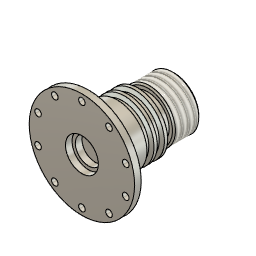
peer challenge (Autodesk Fusion 360 design; units mm, degrees)
Autodesk Fusion 360 part; units mm, degrees
sketch "Sketch1" plane through (0, 0, 0) normal (1, 0, 0) x (0, 0, -1)
  line L0 (0, 0) -> (0, 50.8)
  line L1 (0, 50.8) -> (6.35, 50.8)
  line L2 (6.35, 50.8) -> (6.35, 31.75)
  line L3 (6.35, 31.75) -> (9.525, 28.575)
  line L4 (9.525, 28.575) -> (34.1224, 28.575)
  line L5 (34.1224, 28.575) -> (35.9555, 25.4)
  line L6 (35.9555, 25.4) -> (39.1305, 25.4)
  line L7 (39.1305, 25.4) -> (40.9636, 28.575)
  line L8 (40.9636, 28.575) -> (44.1386, 28.575)
  line L9 (44.1386, 28.575) -> (45.9717, 25.4)
  line L10 (45.9717, 25.4) -> (49.1467, 25.4)
  line L11 (49.1467, 25.4) -> (50.9798, 28.575)
  line L12 (50.9798, 28.575) -> (54.1548, 28.575)
  line L13 (54.1548, 28.575) -> (58.7375, 20.6375)
  line L14 (58.7375, 20.6375) -> (63.5, 20.6375)
  line L15 (63.5, 20.6375) -> (63.5, 25.4)
  line L16 (63.5, 25.4) -> (88.9, 25.4)
  line L17 (88.9, 25.4) -> (88.9, 15.875)
  line L18 (88.9, 15.875) -> (85.725, 15.875)
  line L19 (85.725, 15.875) -> (85.725, 17.4625)
  line L20 (85.725, 17.4625) -> (82.55, 17.4625)
  line L21 (82.55, 17.4625) -> (82.55, 15.875)
  line L22 (82.55, 15.875) -> (76.2, 15.875)
  line L23 (76.2, 15.875) -> (76.2, 12.7)
  line L24 (76.2, 12.7) -> (63.5, 12.7)
  line L25 (63.5, 12.7) -> (63.5, 0)
  line L26 (63.5, 0) -> (12.7, 0)
  line L27 (12.7, 0) -> (12.7, 12.7)
  line L28 (12.7, 12.7) -> (6.35, 12.7)
  line L29 (6.35, 12.7) -> (6.35, 15.875)
  line L30 (6.35, 15.875) -> (0, 15.875)
  dimension "d1" = 6.35
  dimension "d2" = 45
  dimension "d3" = 3.175
  dimension "d4" = 57.15
  dimension "d5" = 3.175
  dimension "d6" = 60
  dimension "d7" = 60
  dimension "d8" = 60
  dimension "d9" = 60
  dimension "d10" = 60
  dimension "d11" = 4.7625
  dimension "d12" = 50.8
  dimension "d13" = 12.7
  dimension "d14" = 25.4
  dimension "d15" = 31.75
  dimension "d16" = 6.35
  dimension "d17" = 3.175
  dimension "d18" = 3.175
  dimension "d19" = 34.925
  dimension "d20" = 88.9
  dimension "d21" = 25.4
  dimension "d22" = 12.7
  dimension "d23" = 25.4
  dimension "d24" = 41.275
  dimension "d25" = 3.175
  dimension "d26" = 101.6
  constraint coincident L0.start origin
  constraint vertical L0
  constraint perpendicular L0 L1
  constraint perpendicular L1 L2
  constraint perpendicular L0 L4
  constraint parallel L4 L6
  constraint parallel L6 L8
  constraint parallel L6 L10
  constraint parallel L6 L12
  constraint parallel L12 L14
  constraint perpendicular L14 L15
  constraint perpendicular L15 L16
  constraint perpendicular L16 L17
  constraint perpendicular L17 L18
  constraint perpendicular L18 L19
  constraint perpendicular L17 L20
  constraint perpendicular L18 L21
  constraint perpendicular L21 L22
  constraint perpendicular L22 L23
  constraint perpendicular L23 L24
  constraint perpendicular L24 L25
  constraint perpendicular L25 L26
  constraint perpendicular L26 L27
  constraint perpendicular L27 L28
  constraint perpendicular L28 L29
  constraint perpendicular L29 L30
  constraint collinear L4 L8
  constraint collinear L8 L12
  constraint equal L8 L12
  constraint equal L6 L10
  constraint equal L6 L8
  constraint collinear L6 L10
  constraint coincident L0.start L26
  constraint coincident L0 L30.end
  constraint collinear L24 L28
  constraint collinear L22 L30
  constraint collinear L18 L22
  measures "d1" distance of L0.end L1.end
  measures "d2" angle of L2 L3
  measures "d3" horizontal distance of L2.end L3.end
  measures "d5" distance of L5.end L6.end
  measures "d6" angle of L5 L6
  measures "d7" angle of L6 L7
  measures "d8" angle of L9 L10
  measures "d9" angle of L10 L11
  measures "d10" angle of L13 L14
  measures "d11" distance of L13.end L14.end
  measures "d13" distance of L0.start L27
  measures "d16" distance of L29.end L30.end
  measures "d17" distance of L19.end L20.end
  measures "d18" distance of L17.end L18.end
  measures "d20" distance of L0.start L17
  measures "d21" distance of L17 L25
  measures "d22" distance of L17 L23
  measures "d23" distance of L15.end L16.end
  measures "d25" distance of L10 L12
revolve "Revolve1" add sketch "Sketch1" angle 360 about axis through (0, 0, -63.5) along (0, 0, 1)
chamfer "Chamfer1" distance 1.5875 angle 45 3 edges at (-23.6811, 9.185, -63.5) (-23.6811, 9.185, -88.9) (-14.8007, 5.7406, -88.9)
thread "Thread1" "ANSI Unified Screw Threads 2.0 2-4.5 UNC 3A" major diameter 50.5206 minor diameter 44.0766 pitch 6.35 angle 60 resizes the face on face at (20.9839, 14.3121, -72.4958)
sketch "Sketch2" plane through (0, 0, 0) normal (0, 0, 1) x (1, 0, 0)
  circle A0 centre (0, 0) radius 15.875
  circle A1 centre (0, 0) radius 50.8
  circle A2 centre (0, 44.45) radius 3.175
  dimension "d29" = 44.45
  dimension "d30" = 6.35
  constraint vertical A0.centre A2.centre
  measures "d29" distance of A0.centre A2.centre
  measures "d30" diameter of A2
extrude "Extrude1" cut sketch "Sketch2" against normal through all contours A2
pattern_circular "C-Pattern1" count 10 over 360 about axis through (0, 0, 0) along (0, 0, -1) of "Extrude1"
equation "d7 = d6"
equation "d8 = d6"
equation "d9 = d6"
equation "d10 = d6"
